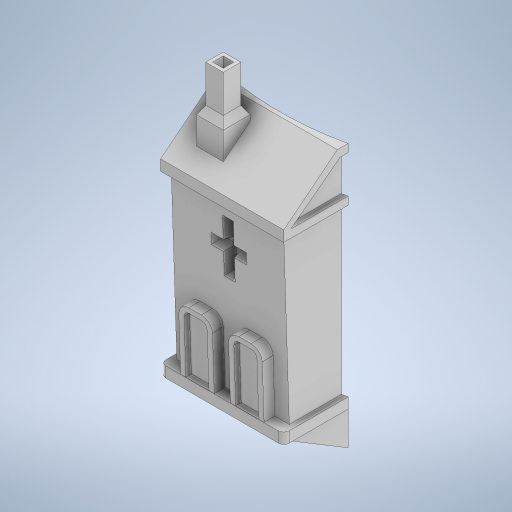
# Autodesk Inventor part: 屋1 物2
Saved by Autodesk Inventor 2024 (Build 280153000, 153)
## iProperties
Created: 2024-05-20
Part Number: 屋1 物2
Material: 一般
Document SubType Name: Modeling
Designer: User
Density: 1 g/cm^3
Appearance: 預設
Author: User
Autodesk Inventor part; units mm, degrees
ref_plane "YZ Plane" through (0, 0, 0) normal (1, 0, 0) x (0, 1, 0)
ref_plane "XZ Plane" through (0, 0, 0) normal (0, 1, 0) x (-1, 0, 0)
ref_plane "XY Plane" through (0, 0, 0) normal (0, 0, 1) x (1, 0, 0)
sketch "草圖1" plane through (0, 0, 0) normal (1, 0, 0) x (0, 1, 0)
  line L0 (10, 0) -> (10, 2)
  line L1 (0, 0) -> (0, 12)
  line L2 (10, 0) -> (0, 0)
  line L3 (0, 12) -> (2, 12)
  line L4 (2, 12) -> (10, 2)
  dimension "d0" = 2
  dimension "d1" = 12
  dimension "d2" = 10
  dimension "d3" = 2
  constraints: 10 end point, 2 horizontal, 2 vertical
  measures "d0" distance of L0.start L0.end
  measures "d1" distance of L1.start L1.end
  measures "d2" distance of L0.start L1.start
  measures "d3" distance of L1.end L3.end
extrude "擠出1" add sketch "草圖1" along normal blind 23
sketch "草圖2" plane through (0, 0, 0) normal (0, -1, 0) x (1, 0, 0)
  line L0 (0, 0) -> (23, 0) projected
  line L1 (1, 0) -> (22, 0)
  line L2 (22, 0) -> (22, 11)
  line L3 (22, 11) -> (1, 11)
  line L4 (1, 11) -> (1, 0)
  line L5 (23, 12) -> (23, 0) projected
  line L6 (0, 12) -> (0, 0) projected
  point P0 (23, 6)
  point P1 (0, 6)
  dimension "d6" = 11
  dimension "d7" = 21
  dimension "d8" = 1
  dimension "d9" = 1
  constraints: 8 end point, 2 midpoint, 2 parallel, 1 horizontal, 1 perpendicular, 1 point on line
  measures "d6" distance of L1.end L2.end
  measures "d7" distance of L2.end L3.end
  measures "d8" distance from line of point (23, 6) L2
  measures "d9" distance from line of point (0, 6) L4
extrude "擠出2" add sketch "草圖2" along normal blind 31
sketch "草圖3" plane through (1, 0, 0) normal (-1, 0, 0) x (0, 0, 1)
  line L0 (12, 0) -> (0, 0)
  line L1 (11, 0) -> (11, -31)
  line L2 (11, 0) -> (9.971867, -30.982946)
  line L3 (9.971867, -30.982946) -> (0, -30.982946)
  line L4 (0, 0) -> (0, -31)
  line L5 (0, -31) -> (11, -31)
  line L6 (0, -30.982946) -> (0, -31)
  line L7 (0, -31) -> (11, -31)
  line L8 (11, -31) -> (11, 0)
  dimension "d13" = 31
  constraints: 10 end point, 1 horizontal, 1 parallel, 1 perpendicular, 1 point on line, 1 vertical
  measures "d13" distance of L1.start L2.end
extrude "擠出3" cut sketch "草圖3" against normal up to next contours L1 L5 L4 L3 L2
sketch "草圖4" plane through (0, 0, 0) normal (0, -1, 0) x (1, 0, 0)
  line L0 (3.7, 9) -> (8.7, 9)
  line L1 (8.7, 9) -> (8.7, 4)
  line L2 (8.7, 4) -> (3.7, 4)
  line L3 (3.7, 4) -> (3.7, 9)
  line L4 (0, 12) -> (23, 12) projected
  line L5 (0, 12) -> (0, 0) projected
  dimension "d16" = 3
  dimension "d17" = 3.7
  dimension "d18" = 5
  dimension "d19" = 5
  constraints: 8 end point, 2 parallel, 1 horizontal, 1 perpendicular
  measures "d16" distance between parallel lines of L4 L0
  measures "d17" distance between parallel lines of L5 L3
  measures "d18" distance of L0.start L0.end
  measures "d19" distance of L0.end L1.end
extrude "擠出4" add sketch "草圖4" against normal blind 9.5
sketch "草圖5" plane through (0, 9.5, 0) normal (0, 1, 0) x (1, 0, 0)
  line L0 (8.7, -4) -> (3.7, -4) projected
  line L1 (8.7, -9) -> (3.7, -9) projected
  line L2 (3.7, -4) -> (8.7, -4)
  line L3 (8.7, -4) -> (8.7, -9)
  line L4 (8.7, -9) -> (3.7, -9)
  line L5 (3.7, -9) -> (3.7, -4)
  point P0 (0, 0)
  constraints: 8 end point, 2 parallel, 1 horizontal, 1 perpendicular
extrude "擠出5" add sketch "草圖5" along normal blind 1.5 draft -30
sketch "草圖6" plane through (0, 11, 0) normal (0, 1, 0) x (1, 0, 0)
  line L0 (4.566025, -8.133975) -> (4.566025, -4.866025)
  line L1 (7.833975, -4.866025) -> (7.833975, -8.133975)
  line L2 (4.566025, -8.133975) -> (7.833975, -8.133975)
  line L3 (7.833975, -8.133975) -> (7.833975, -4.866025)
  line L4 (7.833975, -4.866025) -> (4.566025, -4.866025)
  line L5 (4.566025, -4.866025) -> (4.566025, -8.133975)
  point P0 (0, 0)
  constraints: 8 end point, 2 parallel, 1 horizontal, 1 perpendicular
extrude "擠出6" add sketch "草圖6" along normal blind 7
sketch "草圖7" plane through (1, 0, 11) normal (0, -0.0331656, 0.9994499) x (1, 0, 0)
  line L0 (9.5, -2.366834) -> (11.5, -2.366834)
  line L1 (11.5, -2.366834) -> (11.5, -12.366834)
  line L2 (11.5, -12.366834) -> (9.5, -12.366834)
  line L3 (9.5, -12.366834) -> (9.5, -2.366834)
  line L4 (7.2, -6.366834) -> (13.8, -6.366834)
  line L5 (13.8, -6.366834) -> (13.8, -8.366834)
  line L6 (13.8, -8.366834) -> (7.2, -8.366834)
  line L7 (7.2, -8.366834) -> (7.2, -6.366834)
  line L8 (-1, 0.033166) -> (22, 0.033166)
  line L9 (0, -31) -> (0, 0)
  line L10 (21, 0) -> (21, -31)
  point P0 (-1, -0.364821)
  point P1 (9.5, -8.366834)
  point P2 (11.5, -8.366834)
  point P3 (11.5, -6.366834)
  point P4 (9.5, -6.366834)
  dimension "d26" = 2
  dimension "d27" = 10
  dimension "d28" = 6.6
  dimension "d29" = 2
  dimension "d30" = 2.4
  dimension "d31" = 7.2
  dimension "d32" = 7.2
  dimension "d33" = 9.5
  dimension "d34" = 9.5
  dimension "d35" = 4
  constraints: 16 end point, 4 parallel, 2 horizontal, 2 perpendicular
  measures "d26" distance of L1.end L2.end
  measures "d27" distance of L2.end L0.start
  measures "d28" distance of L5.end L6.end
  measures "d29" distance of L4.end L5.end
  measures "d30" distance between parallel lines of L8 L0
  measures "d31" distance between parallel lines of L9 L7
  measures "d32" distance between parallel lines of L10 L5
  measures "d33" distance between parallel lines of L9 L3
  measures "d34" distance between parallel lines of L10 L1
  measures "d35" distance between parallel lines of L0 L4
sketch "草圖7 outline for 擠出7" plane through (1, 0, 11) normal (0, -0.0331656, 0.9994499) x (1, 0, 0)
  line L0 (7.2, -6.366834) -> (7.2, -8.366834)
  line L1 (9.5, -6.366834) -> (7.2, -6.366834)
  line L2 (9.5, -2.366834) -> (9.5, -6.366834)
  line L3 (11.5, -2.366834) -> (9.5, -2.366834)
  line L4 (11.5, -6.366834) -> (11.5, -2.366834)
  line L5 (13.8, -6.366834) -> (11.5, -6.366834)
  line L6 (13.8, -8.366834) -> (13.8, -6.366834)
  line L7 (11.5, -8.366834) -> (13.8, -8.366834)
  line L8 (11.5, -12.366834) -> (11.5, -8.366834)
  line L9 (9.5, -12.366834) -> (11.5, -12.366834)
  line L10 (9.5, -8.366834) -> (9.5, -12.366834)
  line L11 (7.2, -8.366834) -> (9.5, -8.366834)
extrude "擠出7" cut sketch "草圖7 outline for 擠出7" against normal blind 2 draft -10
sketch "草圖8" plane through (1, -30.982946, 0) normal (0, -1, 0) x (1, 0, 0)
  line L0 (-1, 0) -> (0, 0) projected
  line L1 (22, 2) -> (22, 12) projected
  line L2 (-1, 0) -> (22, 0)
  line L3 (22, 0) -> (22, 11)
  line L4 (21, 12) -> (0, 12)
  line L5 (-1, 11) -> (-1, 0)
  arc A0 (0, 12) -> (-1, 11) centre (0, 11) ccw
  arc A1 (22, 11) -> (21, 12) centre (21, 11) ccw
  point P0 (-1, 12)
  point P1 (22, 2)
  dimension "d40" = 1
  constraints: 8 end point, 4 point on circle, 4 point on line, 4 tangent, 2 centre point, 2 parallel, 1 equal radius, 1 horizontal, 1 perpendicular
  measures "d40" radius of A0
extrude "擠出8" add sketch "草圖8" along normal blind 2
sketch "草圖9" plane through (0, 0, 0) normal (-1, 0, 0) x (0, 0, 1)
  line L0 (2, 10) -> (12, 2)
  line L1 (0, 10) -> (2, 10)
  line L2 (12, 2) -> (12, 0)
  line L3 (12, 0) -> (0, 0)
  line L4 (0, 0) -> (0, 10)
  line L5 (1.473828, 8.5) -> (0, 8.5)
  line L6 (10.5, 1.5) -> (0, 1.5)
  line L7 (1.473828, 8.5) -> (10.5, 1.658737)
  line L8 (10.5, 1.658737) -> (10.5, 1.5)
  dimension "d46" = 1.5
  dimension "d47" = 1.5
  dimension "d48" = 1.5
  dimension "d49" = 1.5
  constraints: 8 end point, 3 perpendicular, 2 point on line
  measures "d46" distance between parallel lines of L3 L6
  measures "d47" distance between parallel lines of L1 L5
  measures "d48" distance between parallel lines of L2 L8
  measures "d49" angle of L0 L7
extrude "擠出9" cut sketch "草圖9" against normal blind 1 contours L5 L7 L8 L6 L4
sketch "草圖10" plane through (23, 0, 0) normal (1, 0, 0) x (0, 0, -1)
  line L0 (0, 0) -> (0, 1.5)
  line L1 (-10.5, 1.5) -> (0, 1.5)
  line L2 (0, 1.5) -> (-10.5, 1.5)
  line L3 (-1.473828, 8.5) -> (-10.5, 1.658737)
  line L4 (-10.5, 1.5) -> (-10.5, 1.658737)
  line L5 (-10.5, 1.658737) -> (-1.473828, 8.5)
  line L6 (-1.473828, 8.5) -> (0, 8.5)
  line L7 (0, 0) -> (0, 10)
  line L8 (0, 8.5) -> (0, 1.5)
  constraints: 10 end point, 3 collinear, 1 parallel, 1 perpendicular, 1 point on line
extrude "擠出10" cut sketch "草圖10" against normal blind 1
sketch "草圖11" plane through (0, 18, 0) normal (0, 1, 0) x (1, 0, 0)
  line L0 (7.199975, -5.499975) -> (5.199975, -5.499975)
  line L1 (5.199975, -5.499975) -> (5.199975, -7.499975)
  line L2 (5.199975, -7.499975) -> (7.199975, -7.499975)
  line L3 (7.199975, -7.499975) -> (7.199975, -5.499975)
  line L4 (7.833975, -8.133975) -> (7.833975, -4.866025)
  line L5 (4.566025, -4.866025) -> (4.566025, -8.133975)
  line L6 (4.566025, -8.133975) -> (7.833975, -8.133975)
  line L7 (7.833975, -4.866025) -> (4.566025, -4.866025)
  point P0 (0, 0)
  dimension "d54" = 2
  dimension "d55" = 2
  dimension "d58" = 0.634
  dimension "d59" = 0.63395
  dimension "d60" = 0.634
  dimension "d61" = 0.63395
  constraints: 8 end point, 2 parallel, 1 horizontal, 1 perpendicular
  measures "d54" distance of L2.end L0.start
  measures "d55" distance of L0.start L0.end
  measures "d58" distance between parallel lines of L4 L3
  measures "d59" distance between parallel lines of L5 L1
  measures "d60" distance between parallel lines of L6 L2
  measures "d61" distance between parallel lines of L7 L0
extrude "擠出11" cut sketch "草圖11" against normal blind 15 contours L3 L2 L1 L0
sketch "草圖12" plane through (1, 0, 11) normal (0, -0.0331656, 0.9994499) x (1, 0, 0)
  line L0 (0, -31) -> (21, -31) projected
  line L1 (2.7, -31) -> (9, -31)
  line L2 (9, -31) -> (9, -21)
  line L3 (7, -19) -> (4.7, -19)
  line L4 (2.7, -21) -> (2.7, -31)
  line L5 (12, -31) -> (18.3, -31)
  line L6 (18.3, -31) -> (18.3, -21)
  line L7 (16.3, -19) -> (14, -19)
  line L8 (12, -21) -> (12, -31)
  line L9 (0, -31) -> (0, 0) projected
  line L10 (21, 0) -> (21, -31) projected
  arc A0 (4.7, -19) -> (2.7, -21) centre (4.7, -21) ccw
  arc A1 (9, -21) -> (7, -19) centre (7, -21) ccw
  arc A2 (14, -19) -> (12, -21) centre (14, -21) ccw
  arc A3 (18.3, -21) -> (16.3, -19) centre (16.3, -21) ccw
  point P0 (-1, -0.364821)
  point P1 (9, -19)
  point P2 (2.7, -19)
  point P3 (18.3, -19)
  point P4 (12, -19)
  point P5 (12, -31)
  point P6 (18.3, -31)
  point P7 (9, -31)
  dimension "d66" = 6.3
  dimension "d67" = 12
  dimension "d68" = 6.3
  dimension "d69" = 12
  dimension "d70" = 3
  dimension "d71" = 2.7
  dimension "d72" = 2.7
  dimension "d73" = 2
  constraints: 16 end point, 10 point on line, 8 point on circle, 8 tangent, 4 centre point, 4 parallel, 3 equal radius, 2 horizontal, 2 perpendicular
  measures "d66" distance of point (2.7, -19) point (9, -19)
  measures "d67" distance of point (9, -19) L1.end
  measures "d68" distance of point (12, -19) point (18.3, -19)
  measures "d69" distance of point (18.3, -19) L5.end
  measures "d70" distance between parallel lines of L8 L2
  measures "d71" distance between parallel lines of L9 L4
  measures "d72" distance between parallel lines of L10 L6
  measures "d73" radius of A0
extrude "擠出12" add sketch "草圖12" along normal blind 2
sketch "草圖13" plane through (1, -0.066331, 12.9989) normal (0, -0.0331656, 0.9994499) x (1, 0, 0)
  line L0 (9, -30.933632) -> (2.7, -30.933632)
  line L1 (2.7, -30.933632) -> (9, -30.933632)
  line L2 (9, -30.933632) -> (9, -20.933632)
  line L3 (7, -18.933632) -> (4.7, -18.933632)
  line L4 (2.7, -20.933632) -> (2.7, -30.933632)
  line L5 (18.3, -30.933632) -> (12, -30.933632)
  line L6 (12, -30.933632) -> (18.3, -30.933632)
  line L7 (18.3, -30.933632) -> (18.3, -20.933632)
  line L8 (16.3, -18.933632) -> (14, -18.933632)
  line L9 (12, -20.933632) -> (12, -30.933632)
  arc A0 (4.7, -18.933632) -> (2.7, -20.933632) centre (4.7, -20.933632) ccw
  arc A1 (9, -20.933632) -> (7, -18.933632) centre (7, -20.933632) ccw
  arc A2 (14, -18.933632) -> (12, -20.933632) centre (14, -20.933632) ccw
  arc A3 (18.3, -20.933632) -> (16.3, -18.933632) centre (16.3, -20.933632) ccw
  line L10 (4.7, -19.933632) -> (7, -19.933632)
  arc A4 (8, -20.933632) -> (7, -19.933632) centre (7, -20.933632) ccw
  line L11 (8, -20.933632) -> (8, -29.933632)
  line L12 (8, -29.933632) -> (3.7, -29.933632)
  line L13 (3.7, -29.933632) -> (3.7, -20.933632)
  arc A5 (4.7, -19.933632) -> (3.7, -20.933632) centre (4.7, -20.933632) ccw
  line L14 (13, -20.933632) -> (13, -29.933632)
  line L15 (13, -29.933632) -> (17.3, -29.933632)
  line L16 (17.3, -29.933632) -> (17.3, -20.933632)
  arc A6 (17.3, -20.933632) -> (16.3, -19.933632) centre (16.3, -20.933632) ccw
  line L17 (16.3, -19.933632) -> (14, -19.933632)
  arc A7 (14, -19.933632) -> (13, -20.933632) centre (14, -20.933632) ccw
  line L18 (3.7, -29.933632) -> (3.7, -30.933632)
  line L19 (8, -29.933632) -> (8, -30.933632)
  line L20 (13, -29.933632) -> (13, -30.933632)
  line L21 (17.3, -29.933632) -> (17.3, -30.933632)
  point P0 (-1, -0.364821)
  point P1 (9, -18.933632)
  point P2 (2.7, -18.933632)
  point P3 (18.3, -18.933632)
  point P4 (12, -18.933632)
  point P5 (13, -30.933632)
  point P6 (17.3, -30.933632)
  point P7 (3.7, -30.933632)
  point P8 (8, -30.933632)
  dimension "d79" = 6.3
  dimension "d80" = 12
  dimension "d81" = 6.3
  dimension "d82" = 12
  dimension "d83" = 2
  dimension "d84" = 1
  dimension "d85" = 1
  constraints: 40 end point, 16 point on circle, 12 point on line, 10 parallel, 8 centre point, 8 tangent, 6 perpendicular, 3 equal radius, 2 horizontal, 10 other
  measures "d79" distance of point (2.7, -18.934) point (9, -18.934)
  measures "d80" distance of point (9, -18.934) L1.end
  measures "d81" distance of point (12, -18.934) point (18.3, -18.934)
  measures "d82" distance of point (18.3, -18.934) L6.end
  measures "d83" radius of A0
  measures "d84" distance between parallel lines of L3 L10
  measures "d85" radial gap between concentric circles of A2 A7
extrude "擠出13" cut sketch "草圖13" against normal blind 1 contours L0 L18 L12 L19 | L12 L13 A5 L10 A4 L11 | L5 L20 L15 L21 | L15 L14 A7 L17 A6 L16
sketch "草圖14" plane through (0, 10, 2) normal (0, 1, 0) x (1, 0, 0)
  line L0 (0, 2) -> (23, 2)
  arc A0 (0, 2) -> (23, 2) centre (11.5, 53.737317) ccw
  line L1 (23, 2) -> (0, 2)
  dimension "d88" = 53
  constraints: 2 end point, 2 point on circle, 1 centre point, 1 collinear
  measures "d88" radius of A0
extrude "擠出14" cut sketch "草圖14" against normal up to next
sketch "草圖15" plane through (1, -32.982946, 0) normal (0, -1, 0) x (1, 0, 0)
  line L0 (0, 11) -> (21, 11)
  line L1 (21, 9.971867) -> (21, 0.212177)
  line L2 (0, 11) -> (21, 11)
  line L3 (21, 11) -> (21, -1)
  line L4 (21, -1) -> (0, -1)
  line L5 (0, -1) -> (0, 11)
  point P0 (-1, 0)
  dimension "d91" = 12
  constraints: 8 end point, 2 parallel, 1 horizontal, 1 perpendicular, 1 point on line
  measures "d91" distance of L2.end L3.end
extrude "擠出15" add sketch "草圖15" along normal blind 10
sketch "草圖16" plane through (22, -32.982946, 11) normal (1, 0, 0) x (0, 0, -1)
  line L0 (0, 0) -> (0, -10)
  line L1 (0, 0) -> (12, -7.24934)
  line L2 (12, 0) -> (12, -10)
  line L3 (12, -10) -> (0, -10)
  line L4 (12, -10) -> (0, -10)
  line L5 (0, -10) -> (0, 0)
  point P0 (11, 32.982946)
  point P1 (9, 0)
  constraints: 6 end point, 1 collinear, 1 perpendicular, 2 other
extrude "擠出16" cut sketch "草圖16" against normal up to surface (21 mm away)
sketch "草圖17" plane through (1, -40.232286, -1) normal (0, -0.8559364, 0.5170812) x (1, 0, 0)
  line L0 (21, 0) -> (0, 0)
  line L1 (0, 14.019734) -> (21, 14.019734)
  line L2 (5, 0) -> (8, 0)
  line L3 (8, 0) -> (8, 14.019734)
  line L4 (8, 14.019734) -> (5, 14.019734)
  line L5 (5, 14.019734) -> (5, 0)
  line L6 (13, 0) -> (16, 0)
  line L7 (16, 0) -> (16, 14.019734)
  line L8 (16, 14.019734) -> (13, 14.019734)
  line L9 (13, 14.019734) -> (13, 0)
  line L10 (0, 0) -> (0, 14.019734)
  line L11 (21, 14.019734) -> (21, 0)
  point P0 (-1, 21.659294)
  point P1 (13, 14.019734)
  point P2 (5, 14.019734)
  dimension "d96" = 3
  dimension "d97" = 3
  dimension "d98" = 5
  dimension "d99" = 5
  constraints: 16 end point, 4 parallel, 4 point on line, 2 horizontal, 2 perpendicular
  measures "d96" distance of L4.end L3.end
  measures "d97" distance of L8.end L7.end
  measures "d98" distance between parallel lines of L10 L5
  measures "d99" distance between parallel lines of L11 L7
extrude "擠出17" cut sketch "草圖17" against normal blind 0.5 contours L0 L9 L1 L7 | L0 L5 L1 L3
